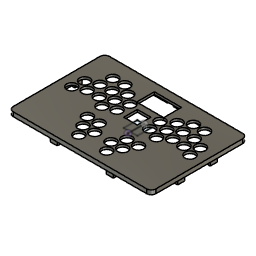
Top (Autodesk Fusion 360 design; units mm, degrees)
Autodesk Fusion 360 part; units mm, degrees
sketch "Sketch1" plane through (0, 0, 0) normal (0, 0, 1) x (1, 0, 0)
  line L0 (-149, 0) -> (-141, 0) construction
  line L1 (67.5, -91) -> (67.5, -99)
  line L2 (52.5, 99) -> (67.5, 99)
  line L3 (-149, -27.5) -> (-141, -27.5)
  line L4 (141, 27.5) -> (141, 42.5)
  line L5 (141, -42.5) -> (141, -27.5)
  line L6 (60, 99) -> (60, 91) construction
  line L7 (-67.5, 91) -> (-67.5, 99)
  line L8 (6.4, 95) -> (6.4, 91)
  line L9 (120, 99) -> (120, 91)
  line L10 (-149, -42.5) -> (-149, -27.5)
  line L11 (-120, -99) -> (-120, -91)
  line L12 (-67.5, -91) -> (-52.5, -91)
  line L13 (-5, 5) -> (5, 5)
  line L14 (149, 42.5) -> (149, 27.5)
  line L15 (141, -27.5) -> (149, -27.5)
  line L16 (0, 103) -> (0, -103) construction
  line L17 (-141, -42.5) -> (-149, -42.5)
  line L18 (141, 0) -> (149, 0) construction
  line L19 (141, 42.5) -> (149, 42.5)
  line L20 (149, -42.5) -> (141, -42.5)
  line L21 (-149, 42.5) -> (-141, 42.5)
  line L22 (149, -70) -> (141, -70)
  line L23 (0, 95) -> (0, 91) construction
  line L24 (5, 5) -> (5, -5)
  line L25 (-67.5, -99) -> (-67.5, -91)
  line L26 (-5, -5) -> (-5, 5)
  line L27 (67.5, -99) -> (52.5, -99)
  line L28 (141, -35) -> (149, -35) construction
  line L29 (-52.5, -91) -> (-52.5, -99)
  line L30 (-5, -5) -> (5, 5) construction
  line L31 (5, -5) -> (-5, -5)
  line L32 (0, -65) -> (0, -75) construction
  line L33 (149, -27.5) -> (149, -42.5)
  line L34 (-6.4, 99) -> (-6.4, 91)
  line L35 (-60, -91) -> (-60, -99) construction
  line L36 (0, 45) -> (0, 35) construction
  line L37 (-67.5, 99) -> (-52.5, 99)
  line L38 (-141, -27.5) -> (-141, -42.5)
  line L39 (-60, 99) -> (-60, 91) construction
  line L40 (52.5, 91) -> (52.5, 99)
  line L41 (-52.5, 91) -> (-67.5, 91)
  line L42 (-149, -35) -> (-141, -35) construction
  line L43 (67.5, 99) -> (67.5, 91)
  line L44 (149, 27.5) -> (141, 27.5)
  line L45 (141, 70) -> (149, 70)
  line L46 (-141, -70) -> (-149, -70)
  line L47 (141, 35) -> (149, 35) construction
  line L48 (120, -91) -> (120, -99)
  line L49 (-6.4, 91) -> (-6.4, 95)
  line L50 (-52.5, -99) -> (-67.5, -99)
  line L51 (5, -5) -> (-5, 5) construction
  line L52 (52.5, -91) -> (67.5, -91)
  line L53 (6.4, 91) -> (-6.4, 91)
  line L54 (-6.4, 95) -> (6.4, 95)
  line L55 (0, -99) -> (0, -91) construction
  line L56 (60, -91) -> (60, -99) construction
  line L57 (-52.5, 99) -> (-52.5, 91)
  line L58 (-149, 70) -> (-141, 70)
  line L59 (120, 91) -> (6.4, 91)
  line L60 (-141, 42.5) -> (-141, 27.5)
  line L61 (-141, -91) -> (-141, 91)
  line L62 (-149, 27.5) -> (-149, 42.5)
  line L63 (6.4, 99) -> (120, 99)
  line L64 (-120, 91) -> (-120, 99)
  line L65 (-141, 91) -> (141, 91)
  line L66 (-141, 27.5) -> (-149, 27.5)
  line L67 (-120, -91) -> (120, -91)
  line L68 (120, -99) -> (-120, -99)
  line L69 (141, -91) -> (-141, -91)
  line L70 (-149, 35) -> (-141, 35) construction
  line L71 (-153, 103) -> (153, 103)
  line L72 (153, -103) -> (-153, -103)
  line L73 (6.4, 91) -> (6.4, 99)
  line L74 (52.5, -99) -> (52.5, -91)
  line L75 (-153, -103) -> (-153, 103)
  line L76 (153, 103) -> (153, -103)
  line L77 (149, 70) -> (149, -70)
  line L78 (-6.4, 91) -> (-120, 91)
  line L79 (-141, 70) -> (-141, -70)
  line L80 (-120, 99) -> (-6.4, 99)
  line L81 (141, -70) -> (141, 70)
  line L82 (-149, -70) -> (-149, 70)
  line L83 (141, 91) -> (141, -91)
  line L84 (67.5, 91) -> (52.5, 91)
  line L85 (-141, -91) -> (141, 91) construction
  line L86 (-153, 0) -> (153, 0) construction
  line L87 (141, -91) -> (-141, 91) construction
  point P0 (0, -70)
  point P1 (130, 80)
  dimension "d119" = 282
  dimension "d120" = 182
  dimension "d121" = 12
  dimension "d122" = 12
  dimension "d123" = 12
  dimension "d124" = 12
  dimension "d125" = 8
  dimension "d126" = 140
  dimension "d127" = 8
  dimension "d128" = 140
  dimension "d129" = 8
  dimension "d130" = 240
  dimension "d131" = 12.8
  dimension "d132" = 4
  dimension "d133" = 15
  dimension "d134" = 15
  dimension "d135" = 15
  dimension "d136" = 15
  dimension "d137" = 15
  dimension "d138" = 15
  dimension "d139" = 15
  dimension "d140" = 15
  dimension "d141" = 35
  dimension "d142" = 35
  dimension "d143" = 35
  dimension "d144" = 35
  dimension "d145" = 60
  dimension "d146" = 60
  dimension "d147" = 113.6
  dimension "d148" = 8
  dimension "d149" = 8
  dimension "d150" = 113.6
  dimension "d181" = 60
  dimension "d182" = 60
  dimension "d191" = 10
  dimension "d192" = 10
  constraint horizontal L69
  constraint perpendicular L61 L69
  constraint parallel L65 L69
  constraint parallel L61 L83
  constraint coincident origin L87
  constraint coincident origin L85
  constraint horizontal L71
  constraint vertical L76
  constraint horizontal L72
  constraint vertical L75
  constraint midpoint L16.start L71
  constraint midpoint L16.end L72
  constraint midpoint L86.start L75
  constraint midpoint L86.end L76
  constraint horizontal L58
  constraint vertical L79
  constraint horizontal L46
  constraint vertical L82
  constraint midpoint L0.start L82
  constraint midpoint L0.end L79
  constraint collinear L0 L86
  constraint horizontal L45
  constraint vertical L77
  constraint horizontal L22
  constraint vertical L81
  constraint midpoint L18.start L81
  constraint midpoint L18.end L77
  constraint collinear L81 L83
  constraint collinear L61 L79
  constraint horizontal L67
  constraint vertical L48
  constraint horizontal L68
  constraint vertical L11
  constraint midpoint L55.start L68
  constraint midpoint L55.end L67
  constraint collinear L16 L55
  constraint collinear L67 L69
  constraint horizontal L54
  constraint vertical L8
  constraint horizontal L53
  constraint vertical L49
  constraint midpoint L23.start L54
  constraint midpoint L23.end L53
  constraint collinear L16 L23
  constraint collinear L53 L65
  constraint horizontal L21
  constraint vertical L60
  constraint horizontal L66
  constraint vertical L62
  constraint midpoint L70.start L62
  constraint midpoint L70.end L60
  constraint horizontal L3
  constraint vertical L38
  constraint horizontal L17
  constraint vertical L10
  constraint midpoint L42.start L10
  constraint midpoint L42.end L38
  constraint horizontal L19
  constraint vertical L14
  constraint horizontal L44
  constraint vertical L4
  constraint midpoint L47.start L4
  constraint midpoint L47.end L14
  constraint horizontal L15
  constraint vertical L33
  constraint horizontal L20
  constraint vertical L5
  constraint midpoint L28.start L5
  constraint midpoint L28.end L33
  constraint midpoint L39.start L37
  constraint midpoint L39.end L41
  constraint midpoint L6.start L2
  constraint midpoint L6.end L84
  constraint midpoint L35.start L12
  constraint midpoint L35.end L50
  constraint midpoint L56.start L52
  constraint midpoint L56.end L27
  constraint collinear L4 L81
  constraint collinear L14 L77
  constraint collinear L33 L77
  constraint collinear L5 L81
  constraint collinear L38 L61
  constraint collinear L10 L82
  constraint collinear L62 L82
  constraint collinear L60 L79
  constraint collinear L50 L68
  constraint collinear L12 L69
  constraint collinear L27 L68
  constraint collinear L52 L67
  constraint horizontal L80
  constraint vertical L34
  constraint horizontal L78
  constraint vertical L64
  constraint collinear L34 L49
  constraint collinear L65 L78
  constraint horizontal L63
  constraint vertical L9
  constraint horizontal L59
  constraint vertical L73
  constraint collinear L8 L73
  constraint collinear L59 L65
  constraint collinear L2 L63
  constraint collinear L65 L84
  constraint collinear L37 L80
  constraint collinear L41 L65
  constraint collinear L16 L32
  constraint collinear L16 L36
  constraint horizontal L31
  constraint perpendicular L26 L31
  constraint parallel L13 L31
  constraint parallel L24 L26
  constraint coincident origin L51
  constraint coincident origin L30
  measures "d119" distance of L61.end L65.end
  measures "d120" distance of L65.end L69.start
  measures "d121" distance of L65 L71
  measures "d122" distance of L76 L83
  measures "d123" distance of L69 L72
  measures "d124" distance of L61 L75
  measures "d125" distance of L58.end L58.start
  measures "d126" distance of L58.start L46.end
  measures "d127" distance of L45.start L45.end
  measures "d128" distance of L45.start L22.end
  measures "d129" distance of L11.start L11.end
  measures "d130" distance of L48.end L11.start
  measures "d131" distance of L8.start L49.end
  measures "d132" distance of L49.end L34.end
  measures "d133" distance of L62.start L21.start
  measures "d134" distance of L10.start L3.start
  measures "d135" distance of L4.start L4.end
  measures "d136" distance of L5.end L5.start
  measures "d137" distance of L37.end L7.end
  measures "d138" distance of L2.end L2.start
  measures "d139" distance of L12.end L12.start
  measures "d140" distance of L1.start L52.start
  measures "d141" distance of L47 L86
  measures "d142" distance of L28 L86
  measures "d143" distance of L70 L86
  measures "d144" distance of L42 L86
  measures "d145" distance of L16 L35
  measures "d146" distance of L16 L56
  measures "d147" distance of L34.start L64.end
  measures "d148" distance of L64.start L64.end
  measures "d149" distance of L9.start L9.end
  measures "d150" distance of L63.start L9.start
  measures "d181" distance of L16 L39
  measures "d182" distance of L6 L16
  measures "d191" distance of L13.start L13.end
  measures "d192" distance of L24.end L13.end
extrude "Extrude1" add sketch "Sketch1" along normal blind 20 contours L1 L27 L52 L67 L68 L69 L74 | L12 L25 L29 L50 L67 L68 L69 | L5 L15 L20 L33 L77 L81 L83 | L4 L14 L19 L44 L77 L81 L83 | L3 L10 L17 L38 L61 L79 L82 | L21 L60 L61 L62 L66 L79 L82 | L2 L40 L43 L59 L63 L65 L84 | L7 L37 L41 L57 L65 L78 L80 makes body 1 at (141, 32.5, 6.6667) makes body 2 at (-149, -37.5, 6.6667) makes body 3 at (-57.5, -99, 6.6667) makes body 4 at (62.5, 91, 6.6667) makes body 5 at (141, -37.5, 6.6667) makes body 6 at (-149, 32.5, 6.6667) makes body 7 at (62.5, -99, 6.6667) makes body 8 at (-62.5, 99, 13.3333)
extrude "Extrude2" add sketch "Sketch1" along normal blind 20 and the other way blind -7.5 contours L1 L48 L67 L68 L69 | L29 L67 L68 L69 L74 | L11 L25 L67 L68 L69 | L20 L22 L77 L81 L83 | L15 L44 L77 L81 L83 | L17 L46 L61 L79 L82 | L19 L45 L77 L81 L83 | L3 L61 L66 L79 L82 | L21 L58 L61 L79 L82 | L9 L43 L59 L63 L65 | L8 L40 L59 L63 L65 L73 | L7 L64 L65 L78 L80 | L34 L49 L57 L65 L78 L80 bodies 1 2 3 4 8 5 6 7
extrude "Extrude3" add sketch "Sketch1" along normal blind 20 and the other way blind -11 contours L71 L72 L75 L76 bodies 1 2 3 4 8
extrude "Extrude4" add sketch "Sketch1" along normal blind 20 and the other way blind -15 contours L4 L5 L12 L38 L41 L52 L53 L59 L60 L61 L65 L67 L69 L78 L79 L81 L83 L84 | L8 L34 L49 L53 L54 L65 L73 bodies 1
extrude "Extrude5" add sketch "Sketch1" along normal blind 20 and the other way blind -11 contours L13 L24 L26 L31 bodies 1
sketch "Sketch2" plane through (0, 0, 0) normal (0, 0, 1) x (1, 0, 0)
  circle A0 centre (0, 0) radius 11
  dimension "d215" = 22
  constraint coincident A0.centre origin
  measures "d215" diameter of A0
extrude "Extrude6" add sketch "Sketch2" along normal blind 20 and the other way blind -15 separate body makes body 9
copy_body "Body->Comp1" bodies 9 removing the originals makes body 10 in component "Button"
sketch "Sketch3" plane through (0, 0, 0) normal (0, 0, 1) x (1, 0, 0)
  line L0 (29, -19) -> (-29, -19)
  line L1 (-29, -19) -> (-29, 19)
  line L2 (-29, 19) -> (29, 19)
  line L3 (29, 19) -> (29, -19)
  line L4 (29, -19) -> (-29, 19) construction
  line L5 (-29, -19) -> (29, 19) construction
  dimension "d220" = 58
  dimension "d221" = 38
  constraint horizontal L0
  constraint perpendicular L0 L1
  constraint parallel L0 L2
  constraint parallel L1 L3
  constraint coincident L4 origin
  constraint coincident L5 origin
  measures "d220" distance of L1.end L2.end
  measures "d221" distance of L0.start L2.end
extrude "Extrude7" add sketch "Sketch3" along normal blind 20 and the other way blind -15 separate body makes body 11
copy_body "Body->Comp2" bodies 11 removing the originals makes body 12 in component "Component"
combine "Combine1" operation cut target body 1 tool bodies 12 body 12 seen with x (1, 0, 0) y (0, 1, 0) z (0, 0, 1) at (0, 66.499, 0)
combine "Combine2" operation cut target body 1 tool bodies 10 10 10 10 10 10 10 10 10 10 10 10 10 10 10 10 10 10 10 10 10 10 10 10 10 10 10 10 10 10 10 10 10 10 10 10 body 10 seen with x (1, 0, 0) y (0, 1, 0) z (0, 0, 1) at (-103.858, 16.162, 0) body 10 seen with x (1, 0, 0) y (0, 1, 0) z (0, 0, 1) at (-58.471, 2.661, 0) body 10 seen with x (1, 0, 0) y (0, 1, 0) z (0, 0, 1) at (-35.111, 11.567, 0) body 10 seen with x (1, 0, 0) y (0, 1, 0) z (0, 0, 1) at (-32.346, 36.414, 0) body 10 seen with x (1, 0, 0) y (0, 1, 0) z (0, 0, 1) at (-126.804, 6.239, 0) body 10 seen with x (1, 0, 0) y (0, 1, 0) z (0, 0, 1) at (58.436, 2.661, 0) body 10 seen with x (1, 0, 0) y (0, 1, 0) z (0, 0, 1) at (126.768, 6.239, 0) body 10 seen with x (1, 0, 0) y (0, 1, 0) z (0, 0, 1) at (-124.039, 31.086, 0) body 10 seen with x (1, 0, 0) y (0, 1, 0) z (0, 0, 1) at (103.822, 16.162, 0) body 10 seen with x (1, 0, 0) y (0, 1, 0) z (0, 0, 1) at (-17.517, -53.915, 0) body 10 seen with x (1, 0, 0) y (0, 1, 0) z (0, 0, 1) at (52.907, 52.355, 0) body 10 seen with x (1, 0, 0) y (0, 1, 0) z (0, 0, 1) at (-101.093, 41.009, 0) body 10 seen with x (1, 0, 0) y (0, 1, 0) z (0, 0, 1) at (124.003, 31.086, 0) body 10 seen with x (1, 0, 0) y (0, 1, 0) z (0, 0, 1) at (-29.856, -75.471, 0) body 10 seen with x (1, 0, 0) y (0, 1, 0) z (0, 0, 1) at (76.075, 41.953, 0) body 10 seen with x (1, 0, 0) y (0, 1, 0) z (0, 0, 1) at (29.82, -75.471, 0) body 10 seen with x (1, 0, 0) y (0, 1, 0) z (0, 0, 1) at (-54.812, -32.147, 0) body 10 seen with x (1, 0, 0) y (0, 1, 0) z (0, 0, 1) at (17.482, -53.915, 0) body 10 seen with x (1, 0, 0) y (0, 1, 0) z (0, 0, 1) at (35.076, 11.567, 0) body 10 seen with x (1, 0, 0) y (0, 1, 0) z (0, 0, 1) at (32.311, 36.414, 0) body 10 seen with x (1, 0, 0) y (0, 1, 0) z (0, 0, 1) at (-73.55, 66.8, 0) body 10 seen with x (1, 0, 0) y (0, 1, 0) z (0, 0, 1) at (-55.706, 27.508, 0) body 10 seen with x (1, 0, 0) y (0, 1, 0) z (0, 0, 1) at (-76.11, 41.953, 0) body 10 seen with x (1, 0, 0) y (0, 1, 0) z (0, 0, 1) at (-42.517, -53.915, 0) body 10 seen with x (1, 0, 0) y (0, 1, 0) z (0, 0, 1) at (54.777, -32.147, 0) body 10 seen with x (1, 0, 0) y (0, 1, 0) z (0, 0, 1) at (98.293, 65.855, 0) body 10 seen with x (1, 0, 0) y (0, 1, 0) z (0, 0, 1) at (42.482, -53.915, 0) body 10 seen with x (1, 0, 0) y (0, 1, 0) z (0, 0, 1) at (78.84, 17.107, 0) body 10 seen with x (1, 0, 0) y (0, 1, 0) z (0, 0, 1) at (-29.812, -32.147, 0) body 10 seen with x (1, 0, 0) y (0, 1, 0) z (0, 0, 1) at (101.057, 41.009, 0) body 10 seen with x (1, 0, 0) y (0, 1, 0) z (0, 0, 1) at (29.777, -32.147, 0) body 10 seen with x (1, 0, 0) y (0, 1, 0) z (0, 0, 1) at (-78.875, 17.107, 0) body 10 seen with x (1, 0, 0) y (0, 1, 0) z (0, 0, 1) at (-98.329, 65.855, 0) body 10 seen with x (1, 0, 0) y (0, 1, 0) z (0, 0, 1) at (-52.942, 52.355, 0) body 10 seen with x (1, 0, 0) y (0, 1, 0) z (0, 0, 1) at (55.671, 27.508, 0) body 10 seen with x (1, 0, 0) y (0, 1, 0) z (0, 0, 1) at (73.514, 66.8, 0)
sketch "Sketch4" plane through (0, 0, 0) normal (0, 0, 1) x (1, 0, 0)
  circle A0 centre (0, 0) radius 2.1
  circle A1 centre (0, 0) radius 1.8
  dimension "d226" = 3.6
  dimension "d227" = 4.2
  constraint coincident A0.centre A1.centre
  constraint concentric A0 A1
  measures "d226" diameter of A1
  measures "d227" diameter of A0
extrude "Extrude8" add sketch "Sketch4" along normal blind 3 separate body makes body 13
extrude "Extrude9" add sketch "Sketch4" along normal blind 4 contours A1 bodies 13
copy_body "Body->Comp3" bodies 13 removing the originals makes body 14 in component "SideHole"
extrude "Extrude12" add sketch "Sketch4" along normal blind 14 and the other way blind -11 separate body makes body 15
extrude "Extrude13" add sketch "Sketch4" along normal blind 15 and the other way blind -11 contours A1 bodies 15
copy_body "Body->Comp5" bodies 15 removing the originals makes body 16 in component "Component'"
combine "Combine5" operation cut target body 1 tool bodies 14 14 16 14 14 14 14 14 14 body 14 seen with x (1, 0, 0) y (0, 1, 0) z (0, 0, 1) at (-60, 95, 0) body 14 seen with x (1, 0, 0) y (0, 1, 0) z (0, 0, 1) at (145, 35, 0) body 14 seen with x (1, 0, 0) y (0, 1, 0) z (0, 0, 1) at (-145, 35, 0) body 14 seen with x (1, 0, 0) y (0, 1, 0) z (0, 0, 1) at (60, 95, 0) body 14 seen with x (1, 0, 0) y (0, 1, 0) z (0, 0, 1) at (-145, -35, 0) body 14 seen with x (1, 0, 0) y (0, 1, 0) z (0, 0, 1) at (-60, -95, 0) body 14 seen with x (1, 0, 0) y (0, 1, 0) z (0, 0, 1) at (145, -35, 0) body 14 seen with x (1, 0, 0) y (0, 1, 0) z (0, 0, 1) at (60, -95, 0)
fillet "Fillet3" radius 10 4 edges at (-153, -103, 15.5) (-153, 103, 15.5) (153, 103, 15.5) (153, -103, 15.5) on bodies 1
sketch "Sketch6" plane through (0, 0, 0) normal (0, 0, 1) x (1, 0, 0)
  line L0 (-14.5, 34.5) -> (14.5, 34.5)
  line L1 (14.5, 34.5) -> (14.5, 5.5)
  line L2 (14.5, 5.5) -> (-14.5, 5.5)
  line L3 (-14.5, 5.5) -> (-14.5, 34.5)
  line L4 (0, 0) -> (0, 35.0077)
  line L5 (0, 34.5) -> (0, 5.5)
  dimension "d261" = 29
  dimension "d262" = 29
  dimension "d263" = 5.5
  constraint horizontal L0
  constraint vertical L1
  constraint horizontal L2
  constraint vertical L3
  constraint coincident L4.start origin
  constraint perpendicular L2 L4
  constraint midpoint L0 L5.start
  constraint midpoint L2 L5.end
  constraint collinear L4 L5
  measures "d261" distance of L0.start L0.end
  measures "d262" distance of L0.end L1.end
  measures "d263" distance of L4.start L2
extrude "Extrude15" add sketch "Sketch6" along normal blind 20 and the other way blind -15 separate body makes body 17
copy_body "Body->Comp7" bodies 17 removing the originals makes body 18 in component "Component''"
combine "Combine6" operation cut target body 1 tool bodies 18
component "Button" placed x (1, 0, 0) y (0, 1, 0) z (0, 0, 1) at (-124.039, 31.086, 0)
component "Button" placed x (1, 0, 0) y (0, 1, 0) z (0, 0, 1) at (-101.093, 41.009, 0)
component "Button" placed x (1, 0, 0) y (0, 1, 0) z (0, 0, 1) at (-76.11, 41.953, 0)
component "Button" placed x (1, 0, 0) y (0, 1, 0) z (0, 0, 1) at (-55.706, 27.508, 0)
component "Button" placed x (1, 0, 0) y (0, 1, 0) z (0, 0, 1) at (-126.804, 6.239, 0)
component "Button" placed x (1, 0, 0) y (0, 1, 0) z (0, 0, 1) at (-103.858, 16.162, 0)
component "Button" placed x (1, 0, 0) y (0, 1, 0) z (0, 0, 1) at (-78.875, 17.107, 0)
component "Button" placed x (1, 0, 0) y (0, 1, 0) z (0, 0, 1) at (-58.471, 2.661, 0)
component "Button" placed x (1, 0, 0) y (0, 1, 0) z (0, 0, 1) at (-98.329, 65.855, 0)
component "Button" placed x (1, 0, 0) y (0, 1, 0) z (0, 0, 1) at (-73.55, 66.8, 0)
component "Button" placed x (1, 0, 0) y (0, 1, 0) z (0, 0, 1) at (-52.942, 52.355, 0)
component "Button" placed x (1, 0, 0) y (0, 1, 0) z (0, 0, 1) at (-32.346, 36.414, 0)
component "Button" placed x (1, 0, 0) y (0, 1, 0) z (0, 0, 1) at (-35.111, 11.567, 0)
component "Button" placed x (1, 0, 0) y (0, 1, 0) z (0, 0, 1) at (-54.812, -32.147, 0)
component "Button" placed x (1, 0, 0) y (0, 1, 0) z (0, 0, 1) at (-29.812, -32.147, 0)
component "Button" placed x (1, 0, 0) y (0, 1, 0) z (0, 0, 1) at (-42.517, -53.915, 0)
component "Button" placed x (1, 0, 0) y (0, 1, 0) z (0, 0, 1) at (-17.517, -53.915, 0)
component "Button" placed x (1, 0, 0) y (0, 1, 0) z (0, 0, 1) at (-29.856, -75.471, 0)
component "Button" placed x (1, 0, 0) y (0, 1, 0) z (0, 0, 1) at (17.482, -53.915, 0)
component "Button" placed x (1, 0, 0) y (0, 1, 0) z (0, 0, 1) at (29.82, -75.471, 0)
component "Button" placed x (1, 0, 0) y (0, 1, 0) z (0, 0, 1) at (42.482, -53.915, 0)
component "Button" placed x (1, 0, 0) y (0, 1, 0) z (0, 0, 1) at (29.777, -32.147, 0)
component "Button" placed x (1, 0, 0) y (0, 1, 0) z (0, 0, 1) at (54.777, -32.147, 0)
component "Button" placed x (1, 0, 0) y (0, 1, 0) z (0, 0, 1) at (58.436, 2.661, 0)
component "Button" placed x (1, 0, 0) y (0, 1, 0) z (0, 0, 1) at (78.84, 17.107, 0)
component "Button" placed x (1, 0, 0) y (0, 1, 0) z (0, 0, 1) at (103.822, 16.162, 0)
component "Button" placed x (1, 0, 0) y (0, 1, 0) z (0, 0, 1) at (126.768, 6.239, 0)
component "Button" placed x (1, 0, 0) y (0, 1, 0) z (0, 0, 1) at (55.671, 27.508, 0)
component "Button" placed x (1, 0, 0) y (0, 1, 0) z (0, 0, 1) at (76.075, 41.953, 0)
component "Button" placed x (1, 0, 0) y (0, 1, 0) z (0, 0, 1) at (101.057, 41.009, 0)
component "Button" placed x (1, 0, 0) y (0, 1, 0) z (0, 0, 1) at (124.003, 31.086, 0)
component "Button" placed x (1, 0, 0) y (0, 1, 0) z (0, 0, 1) at (98.293, 65.855, 0)
component "Button" placed x (1, 0, 0) y (0, 1, 0) z (0, 0, 1) at (73.514, 66.8, 0)
component "Button" placed x (1, 0, 0) y (0, 1, 0) z (0, 0, 1) at (52.907, 52.355, 0)
component "Button" placed x (1, 0, 0) y (0, 1, 0) z (0, 0, 1) at (32.311, 36.414, 0)
component "Button" placed x (1, 0, 0) y (0, 1, 0) z (0, 0, 1) at (35.076, 11.567, 0)
component "Component" placed x (1, 0, 0) y (0, 1, 0) z (0, 0, 1) at (0, 66.499, 0)
component "SideHole" placed x (1, 0, 0) y (0, 1, 0) z (0, 0, 1) at (145, 35, 0)
component "SideHole" placed x (1, 0, 0) y (0, 1, 0) z (0, 0, 1) at (145, -35, 0)
component "SideHole" placed x (1, 0, 0) y (0, 1, 0) z (0, 0, 1) at (-145, 35, 0)
component "SideHole" placed x (1, 0, 0) y (0, 1, 0) z (0, 0, 1) at (-145, -35, 0)
component "SideHole" placed x (1, 0, 0) y (0, 1, 0) z (0, 0, 1) at (60, 95, 0)
component "SideHole" placed x (1, 0, 0) y (0, 1, 0) z (0, 0, 1) at (60, -95, 0)
component "SideHole" placed x (1, 0, 0) y (0, 1, 0) z (0, 0, 1) at (-60, 95, 0)
component "SideHole" placed x (1, 0, 0) y (0, 1, 0) z (0, 0, 1) at (-60, -95, 0)
component "Component'" placed x (1, 0, 0) y (0, 1, 0) z (0, 0, 1) at (0, 0, 0)
component "Component''" placed x (1, 0, 0) y (0, 1, 0) z (0, 0, 1) at (0, 0, 0)
